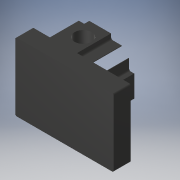
# Autodesk Inventor part: bed_front_cover
Saved by Autodesk Inventor 2018 (Build 220112000, 112)
## iProperties
Created: 2018-05-24
Part Number: bed_front_cover
Material: Plastic, Opaque Black
Document SubType Name: Modeling
Designer: Z. Deniz
Density: 0.952 g/cm^3
Appearance: Smooth - Black
Author: Z. Deniz
Autodesk Inventor part; units mm, degrees
ref_plane "YZ Plane" through (0, 0, 0) normal (1, 0, 0) x (0, 1, 0)
ref_plane "XZ Plane" through (0, 0, 0) normal (0, 1, 0) x (-1, 0, 0)
ref_plane "XY Plane" through (0, 0, 0) normal (0, 0, 1) x (1, 0, 0)
sketch "Sketch2" plane through (0, 0, 0) normal (0, 0, 1) x (1, 0, 0)
  line L0 (0, 0) -> (20, 0)
  line L1 (20, 0) -> (20, 20)
  line L2 (20, 20) -> (0, 20)
  line L3 (0, 20) -> (0, 0)
  line L4 (10, 20) -> (10, 0) construction
  line L5 (0, 10) -> (20, 10) construction
  line L6 (6.8, 18.5) -> (13.2, 18.5)
  line L7 (13.2, 18.5) -> (13.2, 20)
  line L8 (13.2, 20) -> (6.8, 20)
  line L9 (6.8, 20) -> (6.8, 18.5)
  line L10 (6.8, 18.5) -> (13.2, 20) construction
  line L11 (13.2, 18.5) -> (6.8, 20) construction
  line L12 (6.8, 18.5) -> (3.7414, 18.5)
  line L13 (13.2, 18.5) -> (16.2586, 18.5)
  line L14 (3.6707, 18.3293) -> (7.0207, 14.9793)
  line L15 (3.5, 18.5) -> (8.2376, 18.5) construction
  line L16 (7.0914, 14.95) -> (12.9086, 14.95)
  line L17 (16.3293, 18.3293) -> (12.9793, 14.9793)
  line L18 (16.5, 18.5) -> (21.2376, 18.5) construction
  arc A0 (3.7414, 18.5) -> (3.6707, 18.3293) centre (3.7414, 18.4) ccw
  arc A1 (16.3293, 18.3293) -> (16.2586, 18.5) centre (16.2586, 18.4) ccw
  arc A2 (12.9086, 14.95) -> (12.9793, 14.9793) centre (12.9086, 15.05) ccw
  arc A3 (7.0207, 14.9793) -> (7.0914, 14.95) centre (7.0914, 15.05) ccw
  line L19 (20, 20) -> (0, 0) construction
  line L20 (0, 20) -> (20, 0) construction
  line L21 (18.5, 6.8) -> (18.5, 13.2)
  line L22 (18.5, 13.2) -> (20, 13.2)
  line L23 (20, 13.2) -> (20, 6.8)
  line L24 (20, 6.8) -> (18.5, 6.8)
  line L25 (18.5, 6.8) -> (20, 13.2) construction
  line L26 (18.5, 13.2) -> (20, 6.8) construction
  line L27 (18.5, 6.8) -> (18.5, 3.7414)
  line L28 (18.5, 13.2) -> (18.5, 16.2586)
  line L29 (18.3293, 3.6707) -> (14.9793, 7.0207)
  line L30 (18.5, 3.5) -> (18.5, 8.2376) construction
  line L31 (14.95, 7.0914) -> (14.95, 12.9086)
  line L32 (18.3293, 16.3293) -> (14.9793, 12.9793)
  arc A4 (18.3293, 3.6707) -> (18.5, 3.7414) centre (18.4, 3.7414) ccw
  arc A5 (18.5, 16.2586) -> (18.3293, 16.3293) centre (18.4, 16.2586) ccw
  arc A6 (14.9793, 12.9793) -> (14.95, 12.9086) centre (15.05, 12.9086) ccw
  arc A7 (14.95, 7.0914) -> (14.9793, 7.0207) centre (15.05, 7.0914) ccw
  line L33 (1.5, 13.2) -> (1.5, 6.8)
  line L34 (1.5, 6.8) -> (0, 6.8)
  line L35 (0, 6.8) -> (0, 13.2)
  line L36 (0, 13.2) -> (1.5, 13.2)
  line L37 (1.5, 13.2) -> (0, 6.8) construction
  line L38 (1.5, 6.8) -> (0, 13.2) construction
  line L39 (1.5, 13.2) -> (1.5, 16.2586)
  line L40 (1.5, 6.8) -> (1.5, 3.7414)
  line L41 (1.6707, 16.3293) -> (5.0207, 12.9793)
  line L42 (1.5, 16.5) -> (1.5, 11.7624) construction
  line L43 (5.05, 12.9086) -> (5.05, 7.0914)
  line L44 (1.6707, 3.6707) -> (5.0207, 7.0207)
  line L45 (1.5, 3.5) -> (1.5, -1.2376) construction
  arc A8 (1.6707, 16.3293) -> (1.5, 16.2586) centre (1.6, 16.2586) ccw
  arc A9 (1.5, 3.7414) -> (1.6707, 3.6707) centre (1.6, 3.7414) ccw
  arc A10 (5.0207, 7.0207) -> (5.05, 7.0914) centre (4.95, 7.0914) ccw
  arc A11 (5.05, 12.9086) -> (5.0207, 12.9793) centre (4.95, 12.9086) ccw
  line L46 (13.2, 1.5) -> (6.8, 1.5)
  line L47 (13.2, 1.5) -> (6.8, 0) construction
  arc A12 (7.0914, 5.05) -> (7.0207, 5.0207) centre (7.0914, 4.95) ccw
  line L48 (6.8, 1.5) -> (6.8, 0)
  line L49 (6.8, 1.5) -> (3.7414, 1.5)
  line L50 (3.6707, 1.6707) -> (7.0207, 5.0207)
  line L51 (6.8, 0) -> (13.2, 0)
  line L52 (6.8, 1.5) -> (13.2, 0) construction
  line L53 (13.2, 0) -> (13.2, 1.5)
  line L54 (12.9086, 5.05) -> (7.0914, 5.05)
  arc A13 (12.9793, 5.0207) -> (12.9086, 5.05) centre (12.9086, 4.95) ccw
  line L55 (16.5, 1.5) -> (11.7624, 1.5) construction
  arc A14 (16.2586, 1.5) -> (16.3293, 1.6707) centre (16.2586, 1.6) ccw
  arc A15 (3.6707, 1.6707) -> (3.7414, 1.5) centre (3.7414, 1.6) ccw
  line L56 (13.2, 1.5) -> (16.2586, 1.5)
  line L57 (16.3293, 1.6707) -> (12.9793, 5.0207)
  point P0 (10, 19.25)
  point P1 (7.05, 14.95)
  point P2 (12.95, 14.95)
  point P3 (19.25, 10)
  point P4 (18.5, 16.5)
  point P5 (14.95, 7.05)
  point P6 (14.95, 12.95)
  point P7 (0.75, 10)
  point P8 (5.05, 12.95)
  point P9 (5.05, 7.05)
  point P10 (10, 0.75)
  point P11 (7.05, 5.05)
  point P12 (12.95, 5.05)
  point P13 (3.5, 1.5)
  dimension "d23" = 20
  dimension "d24" = 20
  dimension "d25" = 6.4
  dimension "d26" = 1.5
  dimension "d27" = 3.3
  dimension "d28" = 3.3
  dimension "d29" = 45
  dimension "d30" = 135
  dimension "d31" = 5.9
  dimension "d32" = 0.1
  constraints: 116 end point, 67 symmetric about line, 34 point on line, 32 point on circle, 16 centre point, 12 midpoint, 8 tangent, 6 horizontal, 4 parallel, 3 equal radius, 3 perpendicular, 2 equal length, 12 other
  measures "d23" distance of L2.end L1.end
  measures "d24" distance of L1.end L0.end
  measures "d25" distance of L8.end L7.end
  measures "d26" distance between parallel lines of L6 L2
  measures "d27" distance of L6.start L15.start
  measures "d28" distance of L6.end L18.start
  measures "d29" angle of L14 L15
  measures "d30" angle of L17 L18
  measures "d31" distance of point (7.05, 14.95) point (12.95, 14.95)
  measures "d32" radius of A0
extrude "Extrusion3" add sketch "Sketch2" against normal blind 10 contours L48 L46 L53 L0 | L3 L36 L33 L34 | L49 A15 L50 A12 L54 A13 L57 A14 L56 L46 | L33 L39 A8 L41 A11 L43 A10 L44 A9 L40 | L24 L21 L22 L1 | L2 L7 L6 L9 | L27 A4 L29 A7 L31 A6 L32 A5 L28 L21 | L6 L13 A1 L17 A2 L16 A3 L14 A0 L12
extrude "Extrusion4" add sketch "Sketch2" along normal blind 5
sketch "Sketch5" plane through (20, 6.8, -10) normal (1, 0, 0) x (0, 0, -1)
  line L0 (-10, 13.2) -> (-15, 13.2) projected
  line L1 (-15, -6.8) -> (-15, 13.2) projected
  line L2 (-10, 13.2) -> (-15, 13.2)
  line L3 (-15, 13.2) -> (-15, -6.8)
  line L4 (-15, -6.8) -> (-10, -6.8)
  line L5 (-10, -6.8) -> (-10, 13.2)
  point P0 (-10, -6.8)
  constraints: 8 end point, 2 parallel, 1 horizontal, 1 perpendicular
extrude "Extrusion6" add sketch "Sketch5" along normal blind 9
sketch "Sketch6" plane through (6.8, 20, -10) normal (0, 1, 0) x (1, 0, 0)
  circle A0 centre (3.2, -5) radius 2.5
  line L0 (0, -10) -> (0, 0) projected
  line L1 (0, 0) -> (6.4, 0) projected
  point P0 (-6.8, -10)
  dimension "d35" = 5
  dimension "d36" = 3.2
  dimension "d37" = 5
  constraints: 1 centre point
  measures "d35" diameter of A0
  measures "d36" distance from line of L0 A0.centre
  measures "d37" distance from line of A0.centre L1
extrude "Extrusion7" cut sketch "Sketch6" against normal blind 20
sketch "Sketch7" plane through (0, 6.8, -10) normal (-1, 0, 0) x (0, 0, 1)
  circle A0 centre (5, 3.2) radius 2.5
  line L0 (10, 0) -> (0, 0) projected
  line L1 (0, 0) -> (0, 6.4) projected
  point P0 (10, -6.8)
  dimension "d40" = 5
  dimension "d41" = 3.2
  dimension "d42" = 5
  constraints: 1 centre point
  measures "d40" diameter of A0
  measures "d41" distance from line of L0 A0.centre
  measures "d42" distance from line of L1 A0.centre
extrude "Extrusion8" cut sketch "Sketch7" against normal blind 20
fillet "Fillet1" radius 0.5 12 edges at (0, 20, 2.5) (0, 0, 2.5) (29, 0, 2.5) (29, 20, 2.5) (6.8, 18.5, -5) (1.5, 13.2, -5) (13.2, 18.5, -5) (18.5, 13.2, -5) (18.5, 6.8, -5) (13.2, 1.5, -5) (6.8, 1.5, -5) (1.5, 6.8, -5)
body "Solid2"
